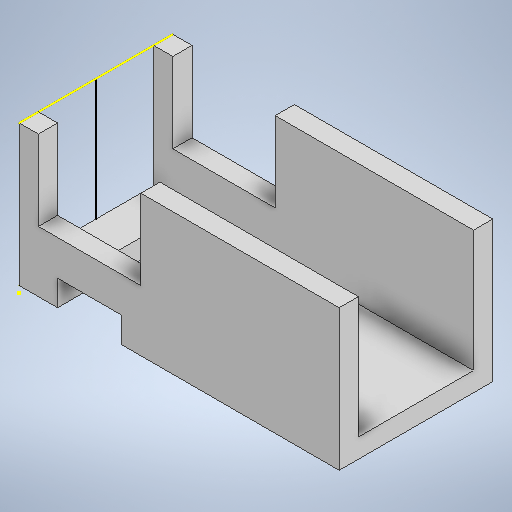
# Autodesk Inventor part: batteryContainer
Saved by Autodesk Inventor 2025.1 (Build 291241020, 241B)
## iProperties
Created: 2025-04-11
Part Number: batteryContainer
Material: Generic
Document SubType Name: Modeling
Designer: omiye
Density: 1 g/cm^3
Appearance: Default
Author: omiye
Autodesk Inventor part; units mm, degrees
ref_plane "YZ Plane" through (0, 0, 0) normal (1, 0, 0) x (0, 1, 0)
ref_plane "XZ Plane" through (0, 0, 0) normal (0, 1, 0) x (-1, 0, 0)
ref_plane "XY Plane" through (0, 0, 0) normal (0, 0, 1) x (1, 0, 0)
sketch "Sketch3" plane through (0, 0, 0) normal (0, 1, 0) x (-1, 0, 0)
  line L0 (0, 0) -> (35, 0)
  line L1 (35, 0) -> (35, -24)
  line L2 (35, -24) -> (0, -24)
  line L3 (0, -24) -> (0, 0)
  dimension "d7" = 35
  dimension "d8" = 24
  constraints: 8 end point, 2 parallel, 1 horizontal, 1 perpendicular
  measures "d7" distance of L1.end L2.end
  measures "d8" distance of L0.end L1.end
extrude "Extrusion2" add sketch "Sketch3" along normal blind 23
sketch "Sketch4" plane through (0, 0, 0) normal (0, -1, 0) x (1, 0, 0)
  line L0 (-35, 0) -> (0, 0) projected
  line L1 (-35, 0) -> (0, 0)
  line L2 (-35, -24) -> (-35, 0) projected
  line L3 (-35, -12) -> (-17.5, -12)
  line L4 (-35, -21) -> (0, -21)
  line L5 (0, -21) -> (0, -3)
  line L6 (0, -3) -> (-35, -3)
  line L7 (-35, -3) -> (-35, -21)
  line L8 (-35, -21) -> (0, -3) construction
  line L9 (0, -21) -> (-35, -3) construction
  dimension "d11" = 35
  dimension "d12" = 18
  constraints: 16 end point, 3 horizontal, 3 midpoint, 2 parallel, 1 perpendicular
  measures "d11" distance of L6.end L5.end
  measures "d12" distance of L5.end L4.end
extrude "Extrusion3" cut sketch "Sketch4" against normal blind 20
sketch "Sketch5" plane through (0, 0, -24) normal (1, 0, 0) x (0, 0, -1)
  line L0 (-21, 0) -> (-24, 0) projected
  line L1 (0, 0) -> (0, 23) projected
  line L2 (-24, 0) -> (0, 0)
  line L3 (0, 0) -> (0, 1)
  line L4 (0, 1) -> (-24, 1)
  line L5 (-24, 1) -> (-24, 0)
  dimension "d15" = 1
  constraints: 8 end point, 2 parallel, 2 perpendicular
  measures "d15" distance of L3.end L1.start
extrude "Extrusion4" cut sketch "Sketch5" against normal blind 50.1625
sketch "Sketch6" plane through (-35, 23, -24) normal (-1, 0, 0) x (0, 0, 1)
  line L0 (3, -22) -> (0, -22) projected
  line L1 (0, -22) -> (3, -22)
  line L2 (3, -22) -> (3, -3)
  line L3 (3, -3) -> (0, -3)
  line L4 (0, -3) -> (0, -22)
  line L5 (24, 0) -> (0, 0) projected
  line L6 (0, -3) -> (24, -3)
  line L7 (24, -3) -> (24, 0)
  line L8 (24, 0) -> (0, 0)
  line L9 (0, 0) -> (0, -3)
  line L10 (24, -22) -> (24, 0) projected
  line L11 (21, -22) -> (21, -3) projected
  line L12 (24, 0) -> (21, 0)
  line L13 (21, 0) -> (21, -22)
  line L14 (21, -22) -> (24, -22)
  line L15 (24, -22) -> (24, 0)
  point P0 (24, -23)
  constraints: 24 end point, 6 parallel, 3 horizontal, 3 perpendicular
extrude "Extrusion5" add sketch "Sketch6" along normal blind 15
sketch "Sketch7" plane through (-50, 23, -24) normal (-1, 0, 0) x (0, 0, 1)
  line L0 (24, 0) -> (0, 0) projected
  line L1 (12, 0) -> (12, -22)
  line L2 (0, 0) -> (0, -22) projected
  line L3 (0, 0) -> (24, 0)
  line L4 (0, -22) -> (3, -22) projected
  line L5 (21, -22) -> (24, -22) projected
  line L6 (0, -22) -> (24, -22)
  point P0 (24, -23)
  constraints: 6 end point, 1 horizontal, 1 midpoint, 1 perpendicular, 1 vertical
sketch "Sketch8" plane through (-50, 23, -24) normal (-1, 0, 0) x (0, 0, 1)
  line L0 (0, -22) -> (3, -22) projected
  line L1 (21, -3) -> (21, -22) projected
  line L2 (3, -22) -> (21, -22)
  line L3 (21, -22) -> (21, -19)
  line L4 (21, -19) -> (3, -19)
  line L5 (3, -19) -> (3, -22)
  point P0 (24, -23)
  dimension "d20" = 3
  constraints: 8 end point, 2 parallel, 1 horizontal, 1 perpendicular, 1 point on line
  measures "d20" distance of L3.end L2.end
extrude "Extrusion6" add sketch "Sketch8" against normal up to surface (50 mm away)
sketch "Sketch9" plane through (0, 23, 0) normal (1, 0, 0) x (0, 0, -1)
  line L0 (3, -19) -> (3, -3) projected
  line L1 (0, 0) -> (24, 0) projected
  line L2 (3, -3) -> (21, -3)
  line L3 (21, -3) -> (21, 0)
  line L4 (21, 0) -> (3, 0)
  line L5 (3, 0) -> (3, -3)
  point P0 (0, -23)
  point P1 (3, 0)
  dimension "d23" = 18
  constraints: 8 end point, 2 parallel, 1 horizontal, 1 perpendicular, 1 point on line
  measures "d23" distance of L4.end L3.end
extrude "Extrusion7" cut sketch "Sketch9" against normal up to surface (50 mm away)
sketch "Sketch10" plane through (0, 1, -24) normal (0, 0, -1) x (-1, 0, 0)
  line L0 (50, 22) -> (50, 3) projected
  line L1 (50, 22) -> (47, 22)
  line L2 (0, 22) -> (50, 22) projected
  line L3 (47, 22) -> (31, 22)
  line L4 (31, 22) -> (31, 9.5)
  line L5 (31, 9.5) -> (47, 9.5)
  line L6 (47, 9.5) -> (47, 22)
  point P0 (0, -1)
  dimension "d26" = 3
  dimension "d27" = 16
  dimension "d28" = 12.5
  constraints: 10 end point, 2 parallel, 1 horizontal, 1 perpendicular, 1 point on line
  measures "d26" distance of L0.start L1.end
  measures "d27" distance of L5.end L4.end
  measures "d28" distance of L4.end L3.end
extrude "Extrusion8" cut sketch "Sketch10" against normal blind 30.6375
sketch "Sketch12" plane through (0, 1, -24) normal (0, 0, -1) x (-1, 0, 0)
  line L0 (31, 9.5) -> (47, 9.5) projected
  line L1 (47, 9.5) -> (39, 9.5)
  line L2 (39, 9.5) -> (39, 0)
  line L3 (50, 0) -> (0, 0) projected
  line L4 (36, 4) -> (42, 4)
  line L5 (42, 4) -> (42, -4)
  line L6 (42, -4) -> (36, -4)
  line L7 (36, -4) -> (36, 4)
  line L8 (36, 4) -> (42, -4) construction
  line L9 (42, 4) -> (36, -4) construction
  line L10 (42, 4) -> (44, 4)
  line L11 (44, 4) -> (44, 0)
  line L12 (44, 0) -> (42, 0)
  line L13 (42, 0) -> (42, 4)
  line L14 (36, 4) -> (34, 4)
  line L15 (34, 4) -> (34, 0)
  line L16 (34, 0) -> (36, 0)
  line L17 (36, 0) -> (36, 4)
  point P0 (0, -1)
  dimension "d34" = 6
  dimension "d35" = 8
  dimension "d36" = 2
  dimension "d37" = 2
  constraints: 32 end point, 6 parallel, 4 perpendicular, 3 midpoint, 3 point on line, 2 horizontal
  measures "d34" distance of L4.start L4.end
  measures "d35" distance of L4.end L5.end
  measures "d36" distance of L11.end L12.end
  measures "d37" distance of L16.end L15.end
extrude "Extrusion10" cut sketch "Sketch12" against normal up to surface (24 mm away) contours L4 L5 L3 L2 | L2 L3 L7 L4 | L7 L3 L15 L14 | L10 L11 L3 L5
body "Solid2"
